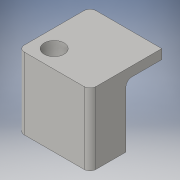
# Autodesk Inventor part: cornerBracketForDLink
Saved by Autodesk Inventor 2016 (Build 200138000, 138)
## iProperties
Created: 2015-10-05
Part Number: cornerBracketForDLink
Material: Generic
Document SubType Name: Modeling
Designer: steele
Density: 1 g/cm^3
Appearance: Default
Author: steele
Autodesk Inventor part; units mm, degrees
ref_plane "YZ Plane" through (0, 0, 0) normal (1, 0, 0) x (0, 1, 0)
ref_plane "XZ Plane" through (0, 0, 0) normal (0, 1, 0) x (-1, 0, 0)
ref_plane "XY Plane" through (0, 0, 0) normal (0, 0, 1) x (1, 0, 0)
sketch "Sketch1" plane through (0, 0, 0) normal (0, 1, 0) x (-1, 0, 0)
  line L0 (-19.05, 19.05) -> (19.05, 19.05)
  line L1 (19.05, 19.05) -> (19.05, -19.05)
  line L2 (19.05, -19.05) -> (-19.05, -19.05)
  line L3 (-19.05, -19.05) -> (-19.05, 19.05)
  line L4 (-19.05, 19.05) -> (19.05, -19.05) construction
  line L5 (19.05, 19.05) -> (-19.05, -19.05) construction
  point P0 (0, 0)
  dimension "width" = 38.1
  dimension "depth" = 38.1
  constraints: 12 end point, 2 midpoint, 2 parallel, 1 horizontal, 1 perpendicular
  measures "width" distance of L0.end L1.end
  measures "depth" distance of L0.start L0.end
extrude "Extrusion1" add sketch "Sketch1" against normal blind 38.1
sketch "Sketch2" plane through (19.05, 0, 19.05) normal (1, 0, 0) x (0, 0, -1)
  line L0 (0, -38.1) -> (38.1, -38.1) projected
  line L1 (38.1, -38.1) -> (19.05, -38.1)
  line L2 (19.05, -38.1) -> (19.05, -5.08)
  line L3 (19.05, -5.08) -> (38.1, -5.08)
  line L4 (38.1, -5.08) -> (38.1, -38.1)
  point P0 (19.05, 0)
  dimension "dLinkHeight" = 33.02
  dimension "dLinkWidth" = 19.05
  constraints: 8 end point, 2 parallel, 1 horizontal, 1 perpendicular
  measures "dLinkHeight" distance of L1.end L2.end
  measures "dLinkWidth" distance between parallel lines of L2 L4
extrude "Extrusion2" cut sketch "Sketch2" against normal blind 19.05
sketch "Sketch6" plane through (0, 0, 0) normal (0, 1, 0) x (1, 0, 0)
  line L0 (19.05, 19.05) -> (19.05, -19.05) construction
  line L1 (19.05, -9.525) -> (-19.05, -9.525) construction
  line L2 (-19.05, -19.05) -> (-19.05, 19.05) construction
  line L3 (-9.525, -19.05) -> (-9.525, 19.05) construction
  line L4 (-19.05, 19.05) -> (19.05, 19.05) construction
  line L5 (19.05, -19.05) -> (-19.05, -19.05) construction
  circle A0 centre (-9.525, -9.525) radius 5.2705
  point P0 (0, 0)
  dimension "widthCenterLine" = 9.525
  dimension "depthCenterLine" = 9.525
  dimension "diamHeadCapScrew" = 10.541
  constraints: 5 point on line, 4 end point, 1 centre point, 1 horizontal, 1 perpendicular
  measures "widthCenterLine" distance between parallel lines of L1 L5
  measures "depthCenterLine" distance between parallel lines of L3 L2
  measures "diamHeadCapScrew" diameter of A0
extrude "Extrusion3" cut sketch "Sketch6" against normal blind 7.62
sketch "Sketch7" plane through (-9.525, -7.62, 9.525) normal (0, 1, 0) x (1, 0, 0)
  circle A0 centre (0, 0) radius 3.302
  point P0 (9.525, 9.525)
  dimension "capScrewThroughHole" = 6.604
  constraints: 1 centre point
  measures "capScrewThroughHole" diameter of A0
extrude "Extrusion4" cut sketch "Sketch7" against normal through all
fillet "Fillet1" radius 3.175 1 edges at (0, -21.59, 0)
fillet "Fillet2" radius 3.175 3 edges at (0.9299, -5.08, -0.9299) (0, -5.08, -11.1125) (11.1125, -5.08, 0)
fillet "Fillet3" radius 3.175 3 edges at (-19.05, -19.05, 19.05) (-19.05, -19.05, -19.05) (19.05, -19.05, 19.05)
equation "\"widthCenterLine\" = -0.5 * dLinkWidth + 0.5 * width"
equation "\"depthCenterLine\" = -0.5 * dLinkWidth + 0.5 * depth"
equation "\"capScrewSpacing\" = 1.016"
equation "\"depthCapScrewSpacing\" = 1.27"
body "Solid1"
